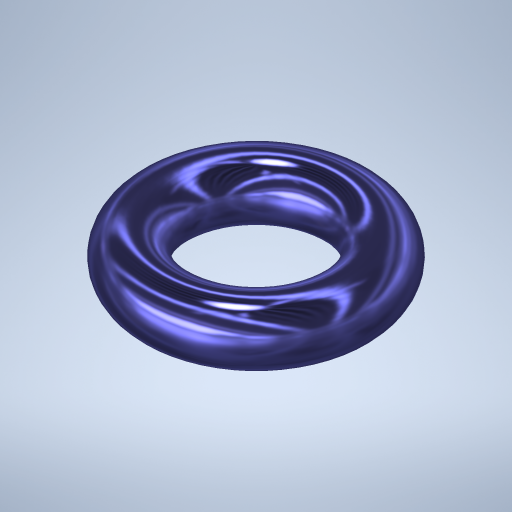
# Autodesk Inventor part: O-Ring
Saved by Autodesk Inventor 2023.1 (Build 271208000, 208)
## iProperties
Created: 2019-11-30
Part Number: O-Ring
Material: Generic
Document SubType Name: Modeling
Designer: Jopa
Density: 1 g/cm^3
Appearance: Bronze - Satin
Author: Jopa
Autodesk Inventor part; units mm, degrees
ref_plane "YZ Plane" through (0, 0, 0) normal (1, 0, 0) x (0, 1, 0)
sketch "Sketch1" plane through (0, 0, 0) normal (0, 0, 1) x (1, 0, 0)
  circle A0 centre (2.3813, 0) radius 0.7938
  line L0 (0, -0.5953) -> (0, 0.5953)
  line L1 (0, 0) -> (2.3813, 0) construction
  dimension "d0" = 1.5875
  dimension "d1" = 2.3813
  constraints: 4 end point, 1 centre point, 1 horizontal, 1 midpoint, 1 perpendicular
  measures "d0" diameter of A0
  measures "d1" distance of L1.start L1.end
revolve "Revolution1" add sketch "Sketch1" angle 360 about axis through (0, -0.5953, 0) along (0, 1, 0)
ref_plane "Work Plane1" through (0, 0.7937, 0) normal (0, 1, 0) x (-1, 0, 0)
ref_plane "Work Plane2" through (0, -0.7937, 0) normal (0, 1, 0) x (-1, 0, 0)
body "Solid1"
